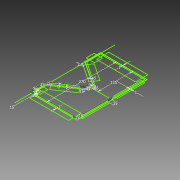
# Autodesk Inventor part: Female
Saved by Autodesk Inventor 2015 (Build 190159000, 159)
## iProperties
Created: 2016-08-08
Part Number: Female
Material: Generic
Document SubType Name: Modeling
Designer: Javier
Density: 1 g/cm^3
Appearance: Default
Author: Javier
Autodesk Inventor part; units mm, degrees
ref_plane "YZ Plane" through (0, 0, 0) normal (1, 0, 0) x (0, 1, 0)
ref_plane "XZ Plane" through (0, 0, 0) normal (0, 1, 0) x (-1, 0, 0)
ref_plane "XY Plane" through (0, 0, 0) normal (0, 0, 1) x (1, 0, 0)
sketch "Sketch1" plane through (0, 0, 0) normal (0, 1, 0) x (-1, 0, 0)
  line L0 (82.171, 116.0061) -> (-97.829, 116.0061)
  line L1 (-97.829, 116.0061) -> (-97.829, -153.9939)
  line L2 (-97.829, -153.9939) -> (82.171, -153.9939)
  line L3 (81.171, 115.0061) -> (-96.829, 115.0061)
  line L4 (-96.829, 115.0061) -> (-96.829, -152.9939)
  line L5 (-96.829, -152.9939) -> (81.171, -152.9939)
  line L6 (81.171, 56.2728) -> (-8.329, -3.7272)
  line L7 (82.171, 55.7393) -> (-7.329, -4.2607)
  line L8 (82.171, -93.7272) -> (-7.329, -33.7272)
  line L9 (81.171, -94.2607) -> (-8.329, -34.2607)
  line L10 (81.171, 56.2728) -> (81.171, 115.0061)
  line L11 (82.171, -153.9939) -> (82.171, -93.7272)
  line L12 (82.171, 55.7393) -> (82.171, 116.0061)
  line L13 (-7.329, -4.2607) -> (-7.329, -33.7272)
  line L14 (-8.329, -3.7272) -> (-8.329, -34.2607)
  line L15 (81.171, -152.9939) -> (81.171, -94.2607)
  line L16 (-92.829, 111.0061) -> (77.171, 111.0061)
  line L17 (-92.829, 111.0061) -> (-92.829, -148.9939)
  line L18 (-92.829, -148.9939) -> (77.171, -148.9939)
  line L19 (-12.329, -1.5931) -> (-12.329, -36.3948)
  line L20 (77.171, 58.4069) -> (-12.329, -1.5931)
  line L21 (77.171, 111.0061) -> (77.171, 58.4069)
  line L22 (77.171, -96.3948) -> (77.171, -148.9939)
  line L23 (77.171, -96.3948) -> (-12.329, -36.3948)
  line L24 (67.171, 133.2815) -> (-82.829, 133.2815)
  line L25 (-82.829, 133.2815) -> (-82.829, 85.6394)
  line L26 (-82.829, 85.6394) -> (67.171, 85.6394)
  line L27 (67.171, 85.6394) -> (67.171, 133.2815)
  line L28 (91.8793, 101.0061) -> (59.7353, 101.0061)
  line L29 (59.7353, 101.0061) -> (59.7353, 70.7393)
  line L30 (59.7353, 70.7393) -> (91.8793, 70.7393)
  line L31 (91.8793, 70.7393) -> (91.8793, 101.0061)
  line L32 (74.0374, 40.9341) -> (7.2402, -3.8462)
  line L33 (56.8116, 66.6293) -> (-9.9856, 21.8491)
  line L34 (56.8116, 66.6293) -> (74.0374, 40.9341)
  line L35 (-9.9856, 21.8491) -> (7.2402, -3.8462)
  line L36 (-88.3298, 101.0061) -> (-103.1355, 101.0061)
  line L37 (-103.1355, 101.0061) -> (-103.1355, -3.9939)
  line L38 (-103.1355, -3.9939) -> (-88.3298, -3.9939)
  line L39 (-88.3298, -3.9939) -> (-88.3298, 101.0061)
  line L40 (-12.329, -18.9939) -> (-92.829, -18.9939)
  line L41 (67.171, -171.2694) -> (-82.829, -171.2694)
  line L42 (-82.829, -171.2694) -> (-82.829, -123.6273)
  line L43 (-82.829, -123.6273) -> (67.171, -123.6273)
  line L44 (67.171, -123.6273) -> (67.171, -171.2694)
  line L45 (91.8793, -138.9939) -> (59.7353, -138.9939)
  line L46 (59.7353, -138.9939) -> (59.7353, -108.7272)
  line L47 (59.7353, -108.7272) -> (91.8793, -108.7272)
  line L48 (91.8793, -108.7272) -> (91.8793, -138.9939)
  line L49 (74.0374, -78.922) -> (7.2402, -34.1417)
  line L50 (56.8116, -104.6172) -> (-9.9856, -59.837)
  line L51 (56.8116, -104.6172) -> (74.0374, -78.922)
  line L52 (-9.9856, -59.837) -> (7.2402, -34.1417)
  line L53 (-88.3298, -138.9939) -> (-103.1355, -138.9939)
  line L54 (-103.1355, -138.9939) -> (-103.1355, -33.9939)
  line L55 (-103.1355, -33.9939) -> (-88.3298, -33.9939)
  line L56 (-88.3298, -33.9939) -> (-88.3298, -138.9939)
  line L57 (79.671, -206.4141) -> (79.671, 178.4349)
  point P0 (0, 0)
  dimension "d0" = 270
  dimension "d3" = 1
  dimension "d4" = 1
  dimension "d5" = 1
  dimension "d17" = 5
  dimension "d18" = 29.4665
  dimension "d28" = 1
  dimension "d29" = 5
  dimension "d30" = 5
  dimension "d31" = 1
  dimension "d32" = 15
  dimension "d33" = 15
  dimension "d34" = 15
  dimension "d35" = 15
  dimension "d36" = 15
  dimension "d37" = 15
  dimension "d38" = 15
  dimension "d39" = 135
  dimension "d40" = 15
  dimension "d41" = 5
  dimension "d42" = 5
  dimension "d48" = 2.5
  constraints: 116 end point, 17 parallel, 16 symmetric about line, 8 perpendicular, 7 horizontal, 5 vertical, 2 midpoint
  measures "d0" distance between parallel lines of L2 L0
  measures "d3" distance between parallel lines of L2 L5
  measures "d4" distance between parallel lines of L1 L4
  measures "d5" distance between parallel lines of L3 L0
  measures "d17" distance between parallel lines of L0 L16
  measures "d18" distance of L7.end L8.end
  measures "d28" distance between parallel lines of L6 L7
  measures "d29" distance between parallel lines of L20 L7
  measures "d30" distance between parallel lines of L21 L12
  measures "d31" distance between parallel lines of L10 L12
  measures "d32" distance from line of L30 L7.start
  measures "d33" distance between parallel lines of L0 L28
  measures "d34" distance between parallel lines of L27 L12
  measures "d35" distance between parallel lines of L1 L25
  measures "d36" distance from line of L7.start L34
  measures "d37" distance from line of L19.start L35
  measures "d38" distance between parallel lines of L36 L0
  measures "d39" distance between parallel lines of L40 L2
  measures "d40" distance between parallel lines of L40 L38
  measures "d41" distance between parallel lines of L8 L23
  measures "d42" distance between parallel lines of L13 L19
  measures "d48" distance between parallel lines of L57 L11
extrude "Extrusion1" add sketch "Sketch1" along normal blind 10 contours L12 L28 L10 L3 L57 L0 | L57 L3 L27 L0 | L12 L30 L10 L28 | L27 L3 L25 L0 | L12 L7 L57 L6 L10 L30 | L25 L3 L4 L36 L1 L0 | L7 L34 L6 L57 | L36 L4 L38 L1 | L7 L35 L6 L34 | L57 L9 L51 L8 | L8 L11 L47 L15 L9 L57 | L38 L4 L55 L1 | L7 L13 L8 L52 L9 L14 L6 L35 | L51 L9 L52 L8 | L55 L4 L53 L1 | L11 L45 L15 L47 | L53 L4 L5 L42 L2 L1 | L11 L2 L57 L5 L15 L45 | L57 L2 L44 L5 | L42 L5 L44 L2
extrude "Extrusion2" add sketch "Sketch1" along normal blind 1 contours L57 L28 L21 L16 L27 L3 | L3 L10 L28 L57 | L10 L30 L57 L28 | L27 L16 L25 L3 | L57 L30 L21 L28 | L10 L6 L57 L30 | L25 L16 L17 L36 L4 L3 | L57 L6 L34 L20 L21 L30 | L36 L17 L38 L4 | L6 L35 L20 L34 | L57 L47 L22 L23 L51 L9 | L9 L15 L47 L57 | L38 L17 L55 L4 | L6 L14 L9 L52 L23 L19 L20 L35 | L51 L23 L52 L9 | L57 L45 L22 L47 | L47 L15 L45 L57 | L55 L17 L53 L4 | L57 L5 L44 L18 L22 L45 | L45 L15 L5 L57 | L53 L17 L18 L42 L5 L4 | L5 L42 L18 L44
extrude "Extrusion3" cut sketch "Sketch1" along normal blind 7.5 contours L28 L31 L30 L12 | L12 L30 L10 L28 | L27 L3 L25 L0 | L0 L25 L24 L27 | L10 L30 L57 L28 | L27 L16 L25 L3 | L57 L30 L21 L28 | L27 L28 L29 L26 L25 L16 | L21 L30 L29 L26 L27 L28 | L36 L4 L38 L1 | L1 L38 L37 L36 | L27 L26 L29 L28 | L34 L32 L35 L7 | L7 L35 L6 L34 | L36 L17 L38 L4 | L6 L35 L20 L34 | L51 L9 L52 L8 | L8 L52 L49 L51 | L55 L4 L53 L1 | L1 L53 L54 L55 | L36 L39 L38 L17 | L20 L35 L33 L34 | L47 L48 L45 L11 | L11 L45 L15 L47 | L51 L23 L52 L9 | L57 L45 L22 L47 | L47 L15 L45 L57 | L55 L17 L53 L4 | L51 L50 L52 L23 | L22 L45 L44 L43 L46 L47 | L55 L56 L53 L17 | L42 L5 L44 L2 | L2 L44 L41 L42 | L45 L46 L43 L44 | L44 L18 L42 L43 L46 L45 | L5 L42 L18 L44
fillet "Fillet1" radius 1 15 edges at (2.9857, 1, -0.1451) (8.329, 1, -18.9939) (-81.171, 1, -101.4939) (-74.171, 1, -152.9939) (-81.171, 1, -145.9939) (-75.1629, 1, 52.2451) (-81.171, 1, 63.5061) (-81.171, 1, 108.0061) (-74.171, 1, 115.0061) (89.829, 1, 115.0061) (96.829, 1, 108.0061) (96.829, 1, -18.9939) (96.829, 1, -145.9939) (2.9857, 1, -37.8428) (89.829, 1, -152.9939)
sketch "Sketch2" plane through (0, 0, 0) normal (0, -1, 0) x (1, 0, 0)
  line L0 (135.8296, -18.9939) -> (-115.0378, -18.9939)
  line L1 (-115.0378, -18.9939) -> (-115.0378, 152.8468)
  line L2 (-115.0378, 152.8468) -> (135.8296, 152.8468)
  line L3 (135.8296, 152.8468) -> (135.8296, -18.9939)
  line L4 (-115.0378, -18.9939) -> (154.388, -18.9939)
  line L5 (154.388, -18.9939) -> (154.388, -183.4288)
  line L6 (154.388, -183.4288) -> (-115.0378, -183.4288)
  line L7 (-115.0378, -183.4288) -> (-115.0378, -18.9939)
  point P0 (0, 0)
  constraints: 16 end point, 4 parallel, 2 horizontal, 2 perpendicular
extrude "Extrusion4" cut sketch "Sketch2" against normal blind 100 contours L0 L1 L2 L3 keep common part
sketch "Sketch4" plane through (97.829, 0, -18.9939) normal (0, 0, -1) x (-1, 0, 0)
  line L0 (0, 0) -> (5, 0)
  line L1 (5, 0) -> (5, 7.5)
  line L2 (5, 7.5) -> (0, 7.5)
  line L3 (0, 7.5) -> (0, 0)
  line L4 (90.5, 0) -> (85.5, 0)
  line L5 (85.5, 0) -> (85.5, 7.5)
  line L6 (85.5, 7.5) -> (90.5, 7.5)
  line L7 (90.5, 7.5) -> (90.5, 0)
  point P0 (97.829, 0)
  dimension "d55" = 5
  dimension "d56" = 5
  dimension "d57" = 7.5
  dimension "d58" = 7.5
  constraints: 16 end point, 4 parallel, 2 horizontal, 2 perpendicular
  measures "d55" distance between parallel lines of L5 L7
  measures "d56" distance between parallel lines of L3 L1
  measures "d57" distance between parallel lines of L0 L2
  measures "d58" distance between parallel lines of L4 L6
extrude "Extrusion6" add sketch "Sketch4" against normal blind 1
body "Solid1"
